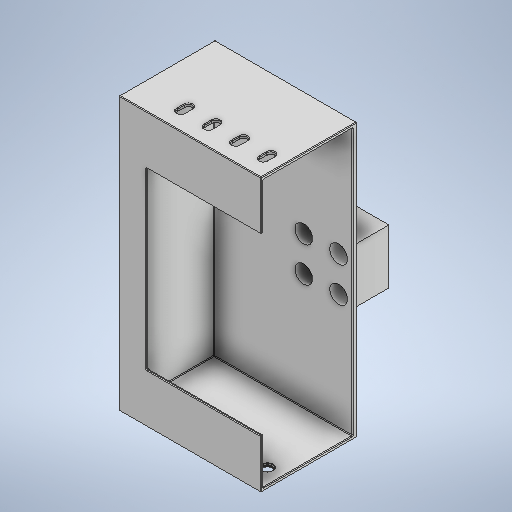
# Autodesk Inventor part: Intake_I2D_Bottom
Saved by Autodesk Inventor 2025 (Build 290162010, 162A)
## iProperties
Created: 2024-10-13
Part Number: Intake_I2D_Bottom
Material: Generic
Document SubType Name: Modeling
Designer: dcfam
Density: 1 g/cm^3
Appearance: Default
Author: dcfam
Autodesk Inventor part; units mm, degrees
ref_plane "YZ Plane" through (0, 0, 0) normal (1, 0, 0) x (0, 1, 0)
ref_plane "XZ Plane" through (0, 0, 0) normal (0, 1, 0) x (-1, 0, 0)
ref_plane "XY Plane" through (0, 0, 0) normal (0, 0, 1) x (1, 0, 0)
sketch "Sketch1" plane through (0, 0, 0) normal (0, 0, 1) x (1, 0, 0)
  line L0 (-32.5, -62.5) -> (32.5, -62.5)
  line L1 (32.5, -62.5) -> (32.5, 62.5)
  line L2 (32.5, 62.5) -> (-32.5, 62.5)
  line L3 (-32.5, 62.5) -> (-32.5, -62.5)
  line L4 (-32.5, -62.5) -> (32.5, 62.5) construction
  line L5 (32.5, -62.5) -> (-32.5, 62.5) construction
  point P0 (0, 0)
  dimension "d0" = 65
  dimension "d1" = 125
  constraints: 12 end point, 2 midpoint, 2 parallel, 1 horizontal, 1 perpendicular
  measures "d0" distance of L2.end L1.end
  measures "d1" distance of L1.end L0.end
extrude "Extrusion1" add sketch "Sketch1" along normal blind 2
sketch "Sketch2" plane through (0, 0, 2) normal (0, 0, 1) x (1, 0, 0)
  line L0 (32.5, -62.5) -> (32.5, 62.5) projected
  line L1 (32.5, 62.5) -> (-32.5, 62.5) projected
  line L2 (-32.5, 62.5) -> (-32.5, -62.5) projected
  line L3 (-32.5, -62.5) -> (32.5, -62.5) projected
  line L4 (31, 61) -> (-31, 61)
  line L5 (-31, 61) -> (-31, -61)
  line L6 (-31, -61) -> (26, -61)
  line L7 (26, -61) -> (32.5, -61)
  line L8 (32.5, -62.5) -> (32.5, 62.5) projected
  line L9 (32.5, -61) -> (32.5, -62.5)
  line L10 (31, 61) -> (32.5, 61)
  line L11 (32.5, 61) -> (32.5, 62.5)
  line L12 (32.5, 62.5) -> (-32.5, 62.5)
  line L13 (-32.5, 62.5) -> (-32.5, -62.5)
  line L14 (-32.5, -62.5) -> (32.5, -62.5)
  point P0 (0, 0)
  dimension "d4" = 1.5
  constraints: 20 end point, 4 perpendicular, 2 collinear, 2 point on line, 1 horizontal, 2 other
  measures "d4" distance between parallel lines of L3 L6
extrude "Extrusion2" add sketch "Sketch2" along normal blind 42 contours L3 L2 L1 L0 L10 L4 L5 L6 L7
sketch "Sketch3" plane through (0, 0, 44) normal (0, 0, 1) x (1, 0, 0)
  line L0 (-32.5, -62.5) -> (32.5, -62.5) projected
  line L1 (32.5, 62.5) -> (-32.5, 62.5) projected
  line L2 (-32.5, -62.5) -> (32.5, -62.5)
  line L3 (32.5, -62.5) -> (32.5, 62.5)
  line L4 (32.5, 62.5) -> (-32.5, 62.5)
  line L5 (-32.5, 62.5) -> (-32.5, -62.5)
  point P0 (0, 0)
  constraints: 8 end point, 2 parallel, 1 horizontal, 1 perpendicular
extrude "Extrusion3" add sketch "Sketch3" against normal blind 1
sketch "Sketch4" plane through (0, 0, 44) normal (0, 0, 1) x (1, 0, 0)
  line L0 (20, -40) -> (-20, -40)
  line L1 (-20, -40) -> (-20, 40)
  line L2 (-20, 40) -> (20, 40)
  line L3 (20, -40) -> (-20, 40) construction
  line L4 (-20, -40) -> (20, 40) construction
  line L5 (20, -40) -> (32.5, -40)
  line L6 (32.5, 61) -> (32.5, -61) projected
  line L7 (20, 40) -> (32.5, 40)
  line L8 (32.5, 40) -> (32.5, -40)
  line L9 (32.5, -40) -> (32.5, 40)
  point P0 (0, 0)
  point P1 (32.5, 40)
  dimension "d9" = 40
  dimension "d10" = 80
  constraints: 18 end point, 3 horizontal, 2 midpoint, 2 perpendicular, 1 collinear, 1 parallel, 1 point on line
  measures "d9" distance of L1.end L2.end
  measures "d10" distance of L0.end L1.end
extrude "Extrusion4" cut sketch "Sketch4" against normal blind 10.525
sketch "Sketch5" plane through (-32.5, 62.5, 0) normal (0, 1, 0) x (1, 0, 0)
  arc A0 (59.7, -32.6288) -> (56.3, -32.6288) centre (58, -32.4292) ccw
  line L0 (56.3, -32.6288) -> (56.3, -35.7388)
  line L1 (56.3, -35.7388) -> (56.3, -32.6288)
  line L2 (56.3, -34.1838) -> (63.0274, -34.1838) construction
  arc A1 (56.3, -35.7388) -> (59.7, -35.7388) centre (58, -35.9383) ccw
  line L3 (58, -35.9383) -> (58, -32.4292) construction
  line L4 (59.7, -32.6288) -> (59.7, -35.7388)
  line L5 (65, 0) -> (65, -44) construction
  line L6 (65, 0) -> (0, 0) construction
  line L7 (0, 0) -> (0, -44) construction
  line L8 (65, -44) -> (0, -44) construction
  arc A2 (43.7, -35.7388) -> (47.1, -35.7388) centre (45.4, -35.9383) ccw
  line L9 (47.1, -32.6288) -> (47.1, -35.7388)
  arc A3 (47.1, -32.6288) -> (43.7, -32.6288) centre (45.4, -32.4292) ccw
  line L10 (43.7, -32.6288) -> (43.7, -35.7388)
  arc A4 (31.1, -35.7388) -> (34.5, -35.7388) centre (32.8, -35.9383) ccw
  line L11 (34.5, -32.6288) -> (34.5, -35.7388)
  arc A5 (34.5, -32.6288) -> (31.1, -32.6288) centre (32.8, -32.4292) ccw
  line L12 (31.1, -32.6288) -> (31.1, -35.7388)
  arc A6 (18.5, -35.7388) -> (21.9, -35.7388) centre (20.2, -35.9383) ccw
  line L13 (21.9, -32.6288) -> (21.9, -35.7388)
  arc A7 (21.9, -32.6288) -> (18.5, -32.6288) centre (20.2, -32.4292) ccw
  line L14 (18.5, -32.6288) -> (18.5, -35.7388)
  line L15 (58, -37.65) -> (20.2, -37.65) construction
  line L16 (39.1, -37.65) -> (39.1, -50.35) construction
  point P0 (32.5, 0)
  point P1 (21.9, -32.6288)
  point P2 (18.5, -35.7388)
  point P3 (21.9, -35.7388)
  point P4 (34.5, -32.6288)
  point P5 (31.1, -35.7388)
  point P6 (34.5, -35.7388)
  point P7 (47.1, -32.6288)
  point P8 (43.7, -35.7388)
  point P9 (47.1, -35.7388)
  point P10 (59.7, -32.6288)
  point P11 (56.3, -35.7388)
  point P12 (59.7, -35.7388)
  dimension "d13" = 3.4
  dimension "d14" = 1.7117
  dimension "d15" = 3.11
  dimension "d16" = 3.11
  dimension "d19" = 12.6
  dimension "d24" = 6.35
  dimension "d37" = 12.7
  dimension "d47" = 32.6288
  dimension "d48" = 1.9726
  dimension "d49" = 1.9726
  dimension "d50" = 35.7388
  dimension "d51" = 1.9726
  dimension "d52" = 35.7388
  dimension "d53" = 5.3726
  dimension "d54" = 32.6288
  dimension "d55" = 14.5726
  dimension "d56" = 35.7388
  dimension "d57" = 14.5726
  dimension "d58" = 35.7388
  dimension "d59" = 17.9726
  dimension "d60" = 32.6288
  dimension "d61" = 27.1726
  dimension "d62" = 35.7388
  dimension "d63" = 27.1726
  dimension "d64" = 35.7388
  dimension "d65" = 30.5726
  dimension "d66" = 32.6288
  dimension "d67" = 39.7726
  dimension "d68" = 35.7388
  dimension "d69" = 39.7726
  dimension "d70" = 35.7388
  dimension "d71" = 43.1726
  dimension "d84" = 5.3
  constraints: 26 end point, 18 point on circle, 8 centre point, 5 symmetric about line, 4 point on line, 3 vertical, 2 horizontal, 2 midpoint, 1 coincident, 1 tangent, 43 other
  measures "d13" distance of A0.start L0.start
  measures "d14" radius of A0
  measures "d15" distance of L0.start L0.end
  measures "d16" distance of L0.end L1.end
  measures "d19" distance of L3.start A2.centre
  measures "d24" distance from line of L8 L15.start
  measures "d37" distance of L16.start L16.end
  measures "d47" distance from line of point (59.7, -32.629) L6
  measures "d49" distance from line of L2.end L5
  measures "d50" distance from line of point (59.7, -35.739) L6
  measures "d52" distance from line of point (56.3, -35.739) L6
  measures "d54" distance from line of point (47.1, -32.629) L6
  measures "d56" distance from line of point (47.1, -35.739) L6
  measures "d58" distance from line of point (43.7, -35.739) L6
  measures "d60" distance from line of point (34.5, -32.629) L6
  measures "d62" distance from line of point (34.5, -35.739) L6
  measures "d64" distance from line of point (31.1, -35.739) L6
  measures "d66" distance from line of point (21.9, -32.629) L6
  measures "d68" distance from line of point (21.9, -35.739) L6
  measures "d70" distance from line of point (18.5, -35.739) L6
  measures "d84" distance between parallel lines of L5 L4
extrude "Extrusion5" cut sketch "Sketch5" against normal blind 25.4
sketch "Sketch6" plane through (-32.5, -62.5, 0) normal (0, -1, 0) x (1, 0, 0)
  circle A0 centre (57.992, 34) radius 1.9625
  line L0 (0, 0) -> (0, 44) projected
  line L1 (0, 0) -> (65, 0) projected
  line L2 (65, 0) -> (65, 44) projected
  line L3 (0, 44) -> (65, 44) projected
  circle A1 centre (49.991, 34) radius 1.9625
  circle A2 centre (41.99, 34) radius 1.9625
  circle A3 centre (33.989, 34) radius 1.9625
  line L4 (33.989, 35.9625) -> (57.992, 35.9625) construction
  line L5 (45.9905, 35.9625) -> (45.9905, 52.0375) construction
  point P0 (32.5, 0)
  dimension "d27" = 3.925
  dimension "d30" = 8.001
  dimension "d35" = 8.0375
  dimension "d36" = 16.075
  dimension "d87" = 7.008
  constraints: 4 end point, 2 centre point, 2 horizontal, 2 vertical alignment, 1 coincident, 1 midpoint, 1 vertical, 10 other
  measures "d30" distance of point (57.992, 34) A1.centre
  measures "d35" distance between parallel lines of L3 L4
  measures "d36" distance of L5.start L5.end
  measures "d87" distance from line of L2 point (57.992, 34)
extrude "Extrusion6" cut sketch "Sketch6" against normal blind 25.4 contours A0 | A1 | A2 | A3
chamfer "Chamfer1" distance 0.5 angle 45 8 edges at (23.5295, -61, 34) (15.5285, -61, 34) (7.5275, -61, 34) (-0.4735, -61, 34) (-0.4735, -62.5, 34) (7.5275, -62.5, 34) (15.5285, -62.5, 34) (23.5295, -62.5, 34)
fillet "Fillet1" radius 0.3 100 edges at (0, -62.5, 44) (15.5285, -61.5, 34) (15.0285, -61, 34) (23.5295, -62, 34) (23.5295, -61.5, 34) (23.0295, -62.5, 34) (7.0275, -62.5, 34) (23.0295, -61, 34) (7.0275, -61, 34) (-0.4735, -62, 34) (-0.4735, -61.5, 34) (-0.9735, -62.5, 34) (-0.9735, -61, 34) (32.5, -61, 22.5) (32.5, -62.5, 22) (0.75, -61, 43) (0.75, -61, 2) (0, -62.5, 0) (-31, -61, 22.5) (-32.5, -62.5, 22) (7.5275, -62, 34) (15.5285, -62, 34) (15.0285, -62.5, 34) (7.5275, -61.5, 34) (-20, 0, 43) (-20, 0, 44) (-31, 0, 43) (-32.5, 0, 44) (-32.5, 0, 0) (0.75, 61, 43) (0.75, 61, 2) (-31, 61, 22.5) (0, 62.5, 44) (0, 62.5, 0) (-32.5, 62.5, 22) (32.5, 61, 22.5) (32.5, 51.25, 44) (32.5, 62.5, 22) (32.5, 50.5, 43) (32.5, -50.5, 43) (32.5, 0, 0) (32.5, 0, 2) (32.5, -51.25, 44) (6.25, -40, 44) (6.25, -40, 43) (32.5, -40, 43.5) (-20, -40, 43.5) (-31, 0, 2) (32.5, 40, 43.5) (-20, 40, 43.5) (6.25, 40, 44) (6.25, 40, 43) (27.2, 62.5, 34.1838) (23.8, 61, 34.1838) (27.2, 61, 34.1838) (25.5, 61, 30.7175) (25.5, 61, 37.65) (23.8, 62.5, 34.1838) (23.8, 61.75, 32.6288) (25.5, 62.5, 30.7175) (27.2, 61.75, 32.6288) (27.2, 61.75, 35.7388) (25.5, 62.5, 37.65) (23.8, 61.75, 35.7388) (-10.6, 62.5, 34.1838) (-10.6, 61, 34.1838) (-14, 61, 34.1838) (-12.3, 61, 30.7175) (-10.6, 61.75, 35.7388) (-10.6, 61.75, 32.6288) (-12.3, 62.5, 30.7175) (-14, 62.5, 34.1838) (-14, 61.75, 32.6288) (-14, 61.75, 35.7388) (-12.3, 62.5, 37.65) (-12.3, 61, 37.65) (14.6, 61, 34.1838) (12.9, 61, 37.65) (11.2, 61, 34.1838) (12.9, 61, 30.7175) (12.9, 62.5, 30.7175) (12.9, 62.5, 37.65) (11.2, 61.75, 35.7388) (11.2, 62.5, 34.1838) (11.2, 61.75, 32.6288) (14.6, 62.5, 34.1838) (14.6, 61.75, 32.6288) (14.6, 61.75, 35.7388) (-1.4, 61, 34.1838) (0.3, 61, 30.7175) (2, 61, 34.1838) (2, 61.75, 35.7388) (2, 61.75, 32.6288) (0.3, 62.5, 30.7175) (-1.4, 61.75, 35.7388) (-1.4, 61.75, 32.6288) (-1.4, 62.5, 34.1838) (0.3, 62.5, 37.65) (2, 62.5, 34.1838) (0.3, 61, 37.65)
sketch "Sketch7" plane through (0, 0, 0) normal (0, 0, -1) x (-1, 0, 0)
  line L0 (-32.2, 62.2) -> (32.2, 62.2) construction
  line L1 (-32.2, -62.2) -> (-32.2, 62.2) construction
  line L2 (32.2, -62.2) -> (-32.2, -62.2) construction
  line L3 (32.2, 62.2) -> (32.2, -62.2) construction
  line L4 (-32.2, 62.2) -> (-32.5, 62.2) construction
  line L5 (-32.5, 62.2) -> (-32.5, -62.2) construction
  line L6 (-32.5, -62.2) -> (-32.2, -62.2) construction
  line L7 (-32.2, -62.2) -> (-32.2, 62.2) construction
  line L8 (32.2, -62.2) -> (32.5, -62.2) construction
  line L9 (32.5, -62.2) -> (32.5, 62.2) construction
  line L10 (32.5, 62.2) -> (32.2, 62.2) construction
  line L11 (32.2, 62.2) -> (32.2, -62.2) construction
  line L12 (-32.2, -62.2) -> (-32.2, -62.5) construction
  line L13 (-32.2, -62.5) -> (32.2, -62.5) construction
  line L14 (32.2, -62.5) -> (32.2, -62.2) construction
  line L15 (32.2, -62.2) -> (-32.2, -62.2) construction
  line L16 (32.2, 62.2) -> (32.2, 62.5) construction
  line L17 (32.2, 62.5) -> (-32.2, 62.5) construction
  line L18 (-32.2, 62.5) -> (-32.2, 62.2) construction
  line L19 (-32.2, 62.2) -> (32.2, 62.2) construction
  line L20 (-32.5, 0) -> (32.5, 0) construction
  line L21 (0, 62.5) -> (0, -62.5) construction
  line L22 (-30.6, 12.5) -> (-5.6, 12.5)
  line L23 (-5.6, 12.5) -> (-5.6, -12.5)
  line L24 (-5.6, -12.5) -> (-30.6, -12.5)
  line L25 (-30.6, -12.5) -> (-30.6, 12.5)
  line L26 (-30.6, 12.5) -> (-5.6, -12.5) construction
  line L27 (-5.6, 12.5) -> (-30.6, -12.5) construction
  point P0 (0, 0)
  point P1 (-18.1, 0)
  dimension "d92" = 25
  dimension "d93" = 25
  dimension "d94" = 38.1
  constraints: 16 end point, 6 midpoint, 2 parallel, 1 horizontal, 1 perpendicular, 1 point on line
  measures "d92" distance of L23.end L24.end
  measures "d93" distance of L22.end L23.end
  measures "d94" distance between parallel lines of L9 L23
extrude "Extrusion7" add sketch "Sketch7" along normal blind 16.5
sketch "Sketch9" plane through (0, 0, -16.5) normal (0, 0, -1) x (-1, 0, 0)
  line L0 (-30.6, -12.5) -> (-5.6, -12.5) projected
  line L1 (-5.6, -12.5) -> (-5.6, 12.5) projected
  line L2 (-5.6, 12.5) -> (-30.6, 12.5) projected
  line L3 (-30.6, 12.5) -> (-30.6, -12.5) projected
  line L4 (-30.6, 0) -> (-5.6, 0) construction
  line L5 (-18.1, 12.5) -> (-18.1, -12.5) construction
  line L6 (-5.6, -12.5) -> (-30.6, 12.5) construction
  line L7 (-30.6, -12.5) -> (-5.6, 12.5) construction
  circle A0 centre (-26.1, -8) radius 2.05
  circle A1 centre (-26.1, 8) radius 2.05
  circle A2 centre (-10.1, -8) radius 2.05
  circle A3 centre (-10.1, 8) radius 2.05
  point P0 (0, 0)
  dimension "d100" = 4.1
  dimension "d101" = 16
  constraints: 8 end point, 4 centre point, 4 midpoint, 3 symmetric about line, 1 perpendicular, 1 point on line, 3 other
  measures "d100" diameter of A0
  measures "d101" distance of A3.centre A2.centre
extrude "Extrusion8" cut sketch "Sketch9" against normal blind 2540 contours A0 | A1 | A2 | A3
sketch "Sketch10" plane through (0, 0, 2) normal (0, 0, 1) x (1, 0, 0)
  circle A0 centre (10.1, -8) radius 2.05 projected
  circle A1 centre (26.1, -8) radius 2.05 projected
  circle A2 centre (10.1, 8) radius 2.05 projected
  circle A3 centre (26.1, 8) radius 2.05 projected
  circle A4 centre (10.1, -8) radius 4.05
  circle A5 centre (10.1, 8) radius 4.05
  circle A6 centre (26.1, 8) radius 4.05
  circle A7 centre (26.1, -8) radius 4.05
  point P0 (0, 0)
  dimension "d104" = 2
  dimension "d105" = 2
  dimension "d106" = 2
  dimension "d107" = 2
  constraints: 4 centre point
  measures "d104" radial gap between concentric circles of A0 A4
  measures "d105" radial gap between concentric circles of A2 A5
  measures "d106" radial gap between concentric circles of A3 A6
  measures "d107" radial gap between concentric circles of A1 A7
extrude "Extrusion9" cut sketch "Sketch10" against normal blind 6
body "Solid1"
